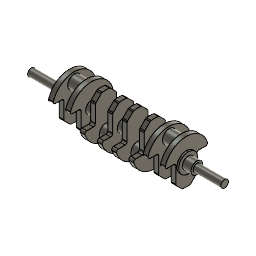
Four Cylinder Engine (Autodesk Fusion 360 archive; units mm, degrees)
design "Crank+Shaft"
Autodesk Fusion 360 part; units mm, degrees
sketch "Sketch1" plane through (0, 0, 0) normal (0, 1, 0) x (1, 0, 0)
  line L0 (0, 0) -> (0, -4)
  line L1 (0, -4) -> (29, -4)
  line L2 (29, -4) -> (29, -6.25)
  line L3 (29, -6.25) -> (38, -6.25)
  line L4 (38, -6.25) -> (38, -10)
  line L5 (38, -10) -> (40, -10)
  line L6 (40, -10) -> (40, 0)
  line L7 (40, 0) -> (0, 0)
  dimension "d1" = 40
  dimension "d2" = 8
  dimension "d3" = 9
  dimension "d4" = 2
  dimension "d5" = 12.5
  dimension "d6" = 20
  constraint coincident L0.start L7.end
  constraint vertical L0
  constraint perpendicular L0 L1
  constraint perpendicular L1 L2
  constraint perpendicular L2 L3
  constraint perpendicular L3 L4
  constraint perpendicular L4 L5
  constraint perpendicular L5 L6
  constraint perpendicular L6 L7
  measures "d1" distance of L6.end L0.start
  measures "d3" distance of L2.end L3.end
  measures "d4" distance of L4.end L5.end
revolve "Revolve1" add sketch "Sketch1" angle 360 about axis through (40, 0, 0) along (-1, 0, 0)
sketch "Sketch2" plane through (40, 0, 0) normal (1, 0, 0) x (0, 1, 0)
  circle A0 centre (0, 0) radius 10
  line L0 (-22.6495, 4) -> (-11, 4)
  line L1 (-11, 4) -> (-11, -16)
  line L2 (-11, -16) -> (-4.4308, -22.5692)
  line L3 (0, 0) -> (0, -30.8331) construction
  line L4 (0, -30.8331) -> (-15.3235, -23.6593) construction
  line L5 (22.6495, 4) -> (11, 4)
  line L6 (11, 4) -> (11, -16)
  line L7 (11, -16) -> (4.4308, -22.5692)
  arc A1 (-4.4308, -22.5692) -> (4.4308, -22.5692) centre (0, 0) ccw
  arc A2 (22.6495, 4) -> (-22.6495, 4) centre (0, 0) ccw
  dimension "d8" = 46
  dimension "d9" = 4
  dimension "d10" = 135
  dimension "d11" = 20
  dimension "d12" = 22
  dimension "d13" = 23
  constraint coincident A0.centre L3.start
  constraint horizontal L0
  constraint perpendicular L0 L1
  constraint vertical L3
  constraint symmetric L0.start L3 L5.start
  constraint symmetric L0.end L3 L5.end
  constraint symmetric L1.end L3 L6.end
  constraint symmetric L2.end L3 L7.end
  constraint concentric A1 A2
  measures "d8" diameter of A1
  measures "d9" distance of A0.centre L0
  measures "d10" angle of L1 L2
  measures "d11" distance of L0.end L1.end
  measures "d12" distance of L1 L6
  measures "d13" radius of A2
extrude "Extrude1" add sketch "Sketch2" along normal blind 5 contours A0 | L0 L1 L2 L5 L6 L7 A1 A2
fillet "Fillet1" radius 2 8 edges at (42.5, -22.6495, 4) (42.5, -11, -16) (42.5, -11, 4) (42.5, -4.4308, -22.5692) (42.5, 22.6495, 4) (42.5, 11, 4) (42.5, 11, -16) (42.5, 4.4308, -22.5692)
sketch "Sketch3" plane through (45, 0, 0) normal (1, 0, 0) x (0, 1, 0)
  arc A0 (3.7876, -22.686) -> (4.8725, -22.1275) centre (3.4583, -20.7133) ccw
  line L0 (4.8725, -22.1275) -> (10.4142, -16.5858)
  arc A1 (10.4142, -16.5858) -> (11, -15.1716) centre (9, -15.1716) ccw
  line L1 (11, -15.1716) -> (11, 2)
  arc A2 (13, 4) -> (11, 2) centre (13, 2) ccw
  line L2 (13, 4) -> (20.1246, 4)
  arc A3 (20.1246, 4) -> (22.0412, 6.5714) centre (20.1246, 6) ccw
  arc A4 (22.0412, 6.5714) -> (-22.0412, 6.5714) centre (0, 0) ccw
  arc A5 (-22.0412, 6.5714) -> (-20.1246, 4) centre (-20.1246, 6) ccw
  line L3 (-20.1246, 4) -> (-13, 4)
  arc A6 (-11, 2) -> (-13, 4) centre (-13, 2) ccw
  line L4 (-11, 2) -> (-11, -15.1716)
  arc A7 (-11, -15.1716) -> (-10.4142, -16.5858) centre (-9, -15.1716) ccw
  line L5 (-10.4142, -16.5858) -> (-4.8725, -22.1275)
  arc A8 (-4.8725, -22.1275) -> (-3.7876, -22.686) centre (-3.4583, -20.7133) ccw
  arc A9 (-3.7876, -22.686) -> (3.7876, -22.686) centre (0, 0) ccw
  circle A10 centre (0, 14) radius 7
  dimension "d18" = 14
  dimension "d19" = 14
  constraint vertical A4.centre A10.centre
  measures "d18" diameter of A10
  measures "d19" distance of A4.centre A10.centre
extrude "Extrude2" add sketch "Sketch3" along normal blind 13 contours A10
pattern_linear "R-Pattern1" count 2 spacing 18 along (1, 0, 0) of "Extrude1", "Fillet1"
sketch "Sketch4" plane through (63, 0, 0) normal (1, 0, 0) x (0, 1, 0)
  arc A0 (3.7876, -22.686) -> (4.8725, -22.1275) centre (3.4583, -20.7133) ccw
  line L0 (4.8725, -22.1275) -> (10.4142, -16.5858)
  arc A1 (10.4142, -16.5858) -> (11, -15.1716) centre (9, -15.1716) ccw
  line L1 (11, -15.1716) -> (11, 2)
  arc A2 (13, 4) -> (11, 2) centre (13, 2) ccw
  line L2 (13, 4) -> (20.1246, 4)
  arc A3 (20.1246, 4) -> (22.0412, 6.5714) centre (20.1246, 6) ccw
  arc A4 (22.0412, 6.5714) -> (-22.0412, 6.5714) centre (0, 0) ccw
  arc A5 (-22.0412, 6.5714) -> (-20.1246, 4) centre (-20.1246, 6) ccw
  line L3 (-20.1246, 4) -> (-13, 4)
  arc A6 (-11, 2) -> (-13, 4) centre (-13, 2) ccw
  line L4 (-11, 2) -> (-11, -15.1716)
  arc A7 (-11, -15.1716) -> (-10.4142, -16.5858) centre (-9, -15.1716) ccw
  line L5 (-10.4142, -16.5858) -> (-4.8725, -22.1275)
  arc A8 (-4.8725, -22.1275) -> (-3.7876, -22.686) centre (-3.4583, -20.7133) ccw
  arc A9 (-3.7876, -22.686) -> (3.7876, -22.686) centre (0, 0) ccw
  circle A10 centre (0, 0) radius 6.25
  dimension "d26" = 12.5
  constraint concentric A4 A10
  measures "d26" diameter of A10
extrude "Extrude3" add sketch "Sketch4" along normal blind 10 contours A10
sketch "Sketch5" plane through (73, 0, 0) normal (1, 0, 0) x (0, 1, 0)
  circle A0 centre (0, 0) radius 6.25
  line L0 (-22.6495, -4) -> (-11, -4)
  line L1 (-11, -4) -> (-11, 16)
  line L2 (-11, 16) -> (-4.4308, 22.5692)
  line L3 (0, 0) -> (0, 36.6926) construction
  line L4 (11, 16) -> (4.4308, 22.5692)
  line L5 (11, -4) -> (11, 16)
  line L6 (22.6495, -4) -> (11, -4)
  arc A1 (-22.6495, -4) -> (22.6495, -4) centre (0, 0) ccw
  arc A2 (4.4308, 22.5692) -> (-4.4308, 22.5692) centre (0, 0) ccw
  dimension "d29" = 46
  dimension "d30" = 135
  dimension "d31" = 20
  dimension "d32" = 11
  dimension "d33" = 4
  dimension "d34" = 23
  constraint coincident A0.centre L3.start
  constraint horizontal L0
  constraint perpendicular L0 L1
  constraint vertical L3
  constraint symmetric L0.start L3 L6.start
  constraint symmetric L0.end L3 L5.start
  constraint symmetric L1.end L3 L4.start
  constraint symmetric L2.end L3 L4.end
  constraint concentric A1 A2
  measures "d29" diameter of A1
  measures "d30" angle of L1 L2
  measures "d31" distance of L0.end L1.end
  measures "d32" distance of A0.centre L1
  measures "d33" vertical distance of A0.centre L0.start
  measures "d34" radius of A2
extrude "Extrude4" add sketch "Sketch5" along normal blind 5 contours A0 | L0 L1 L2 L4 L5 L6 A1 A2
fillet "Fillet2" radius 2 8 edges at (75.5, -11, 16) (75.5, -4.4308, 22.5692) (75.5, -11, -4) (75.5, -22.6495, -4) (75.5, 22.6495, -4) (75.5, 11, -4) (75.5, 11, 16) (75.5, 4.4308, 22.5692)
sketch "Sketch6" plane through (78, 0, 0) normal (1, 0, 0) x (0, 1, 0)
  arc A0 (4.8725, 22.1275) -> (3.7876, 22.686) centre (3.4583, 20.7133) ccw
  arc A1 (3.7876, 22.686) -> (-3.7876, 22.686) centre (0, 0) ccw
  arc A2 (-3.7876, 22.686) -> (-4.8725, 22.1275) centre (-3.4583, 20.7133) ccw
  line L0 (-4.8725, 22.1275) -> (-10.4142, 16.5858)
  arc A3 (-10.4142, 16.5858) -> (-11, 15.1716) centre (-9, 15.1716) ccw
  line L1 (-11, 15.1716) -> (-11, -2)
  arc A4 (-13, -4) -> (-11, -2) centre (-13, -2) ccw
  line L2 (-13, -4) -> (-20.1246, -4)
  arc A5 (-20.1246, -4) -> (-22.0412, -6.5714) centre (-20.1246, -6) ccw
  arc A6 (-22.0412, -6.5714) -> (22.0412, -6.5714) centre (0, 0) ccw
  arc A7 (22.0412, -6.5714) -> (20.1246, -4) centre (20.1246, -6) ccw
  line L3 (20.1246, -4) -> (13, -4)
  arc A8 (11, -2) -> (13, -4) centre (13, -2) ccw
  line L4 (11, -2) -> (11, 15.1716)
  arc A9 (11, 15.1716) -> (10.4142, 16.5858) centre (9, 15.1716) ccw
  line L5 (10.4142, 16.5858) -> (4.8725, 22.1275)
  circle A10 centre (0, -14) radius 7
  dimension "d39" = 14
  dimension "d40" = 14
  constraint vertical A1.centre A10.centre
  measures "d39" diameter of A10
  measures "d40" distance of A1.centre A10.centre
extrude "Extrude5" add sketch "Sketch6" along normal blind 13 contours A10
pattern_linear "R-Pattern2" count 2 spacing 18 along (1, 0, 0) of "Extrude4", "Fillet2"
sketch "Sketch7" plane through (96, 0, 0) normal (1, 0, 0) x (0, 1, 0)
  arc A0 (4.8725, 22.1275) -> (3.7876, 22.686) centre (3.4583, 20.7133) ccw
  arc A1 (3.7876, 22.686) -> (-3.7876, 22.686) centre (0, 0) ccw
  arc A2 (-3.7876, 22.686) -> (-4.8725, 22.1275) centre (-3.4583, 20.7133) ccw
  line L0 (-4.8725, 22.1275) -> (-10.4142, 16.5858)
  arc A3 (-10.4142, 16.5858) -> (-11, 15.1716) centre (-9, 15.1716) ccw
  line L1 (-11, 15.1716) -> (-11, -2)
  arc A4 (-13, -4) -> (-11, -2) centre (-13, -2) ccw
  line L2 (-13, -4) -> (-20.1246, -4)
  arc A5 (-20.1246, -4) -> (-22.0412, -6.5714) centre (-20.1246, -6) ccw
  arc A6 (-22.0412, -6.5714) -> (22.0412, -6.5714) centre (0, 0) ccw
  arc A7 (22.0412, -6.5714) -> (20.1246, -4) centre (20.1246, -6) ccw
  line L3 (20.1246, -4) -> (13, -4)
  arc A8 (11, -2) -> (13, -4) centre (13, -2) ccw
  line L4 (11, -2) -> (11, 15.1716)
  arc A9 (11, 15.1716) -> (10.4142, 16.5858) centre (9, 15.1716) ccw
  line L5 (10.4142, 16.5858) -> (4.8725, 22.1275)
  circle A10 centre (0, 0) radius 6.25
  dimension "d47" = 12.5
  constraint vertical A1.centre A6.centre
  constraint coincident A1.centre A6.centre
  measures "d47" diameter of A10
extrude "Extrude6" add sketch "Sketch7" along normal blind 5 contours A10
mirror "Mirror1" about plane through (101, 0, 0) normal (1, 0, 0) of bodies 1 merged
scale "Scale1" factor 25.4 about (45, -7, 14) bodies 1

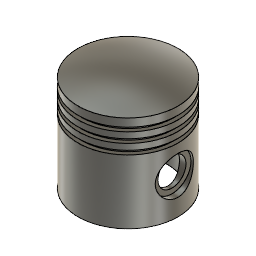
design "Piston (1)"
Autodesk Fusion 360 part; units mm, degrees
sketch "Sketch1" plane through (0, 0, 0) normal (0, 1, 0) x (1, 0, 0)
  line L0 (0, 0) -> (0, -786.4568) construction
  line L1 (0, -660.4) -> (0, -355.6)
  line L2 (0, -355.6) -> (254, -355.6)
  line L3 (254, -355.6) -> (254, 0)
  line L4 (254, 0) -> (317.5, 0)
  line L5 (317.5, 0) -> (317.5, -406.4)
  line L6 (317.5, -406.4) -> (292.1, -406.4)
  line L7 (292.1, -406.4) -> (292.1, -431.8)
  line L8 (292.1, -431.8) -> (317.5, -431.8)
  line L9 (317.5, -431.8) -> (317.5, -469.9)
  line L10 (317.5, -469.9) -> (292.1, -469.9)
  line L11 (292.1, -469.9) -> (292.1, -495.3)
  line L12 (292.1, -495.3) -> (317.5, -495.3)
  line L13 (317.5, -495.3) -> (317.5, -533.4)
  line L14 (317.5, -533.4) -> (292.1, -533.4)
  line L15 (292.1, -533.4) -> (292.1, -558.8)
  line L16 (292.1, -558.8) -> (317.5, -558.8)
  line L17 (317.5, -558.8) -> (317.5, -609.6)
  arc A0 (0, -660.4) -> (317.5, -609.6) centre (0, 357.1875) ccw
  line L18 (0, -660.4) -> (-554.1255, -660.4) construction
  dimension "d1" = 508
  dimension "d2" = 635
  dimension "d3" = 355.6
  dimension "d4" = 406.4
  dimension "d5" = 25.4
  dimension "d6" = 25.4
  dimension "d7" = 38.1
  dimension "d8" = 50.8
  dimension "d22" = 660.4
  constraint coincident L0.start origin
  constraint vertical L0
  constraint coincident L0 L1.start
  constraint coincident L0 L1.end
  constraint perpendicular L0 L2
  constraint perpendicular L2 L3
  constraint perpendicular L3 L4
  constraint perpendicular L4 L5
  constraint perpendicular L3 L6
  constraint perpendicular L6 L7
  constraint perpendicular L7 L8
  constraint perpendicular L8 L9
  constraint perpendicular L9 L10
  constraint perpendicular L10 L11
  constraint perpendicular L11 L12
  constraint perpendicular L12 L13
  constraint perpendicular L13 L14
  constraint perpendicular L14 L15
  constraint perpendicular L15 L16
  constraint perpendicular L16 L17
  constraint horizontal L0.start L3.end
  constraint vertical L5.end L8.end
  constraint vertical L9.end L12.end
  constraint vertical L13.end L16.end
  constraint equal L7 L11
  constraint equal L11 L15
  constraint equal L9 L13
  constraint vertical L7.end L10.end
  constraint vertical L11.end L14.end
  constraint perpendicular L0 L18
  constraint tangent A0 L18
  measures "d3" distance of L2.end L3.end
  measures "d4" distance of L4.end L5.end
  measures "d5" distance of L5.end L6.end
  measures "d6" distance of L6.end L7.end
  measures "d7" distance of L8.end L9.end
  measures "d8" distance of L16.end L17.end
  measures "d22" distance of L0.start L1.start
revolve "Revolve1" add sketch "Sketch1" angle 360 about axis through (0, 0, 0) along (0, 0, 1)
ref_plane "WorkPlane1" through (317.5, 0, 0) normal (1, 0, 0) x (0, 1, 0)
sketch "Sketch2" plane through (317.5, 0, 0) normal (1, 0, 0) x (0, 1, 0)
  circle A0 centre (0, 228.6) radius 120.65
  dimension "d13" = 241.3
  dimension "d14" = 228.6
  constraint vertical origin A0.centre
  measures "d13" diameter of A0
  measures "d14" distance of origin A0.centre
extrude "Extrude1" cut sketch "Sketch2" against normal blind 38.1
sketch "Sketch3" plane through (279.4, 0, 0) normal (1, 0, 0) x (0, 1, 0)
  circle A0 centre (0, 228.6) radius 120.65
  circle A1 centre (0, 228.6) radius 88.9
  dimension "d17" = 177.8
  constraint concentric A0 A1
  measures "d17" diameter of A1
extrude "Extrude2" cut sketch "Sketch3" against normal blind 127 contours A1
mirror "Mirror1" about plane through (0, 0, 0) normal (1, 0, 0) of "Extrude1", "Extrude2"

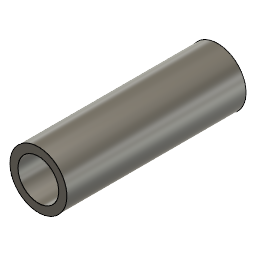
design "piston pin"
part number: 2026-06-25-16-27-55-743
Autodesk Fusion 360 part; units mm, degrees
sketch "Sketch1" plane through (0, 0, 0) normal (0, 0, 1) x (1, 0, 0)
  circle A0 centre (0, 0) radius 63.5
  circle A1 centre (0, 0) radius 88.9
  dimension "d2" = 127
  dimension "d3" = 177.8
  constraint coincident A0.centre A1.centre
  measures "d2" diameter of A0
  measures "d3" diameter of A1
extrude "Extrude1" add sketch "Sketch1" along normal blind 558.8

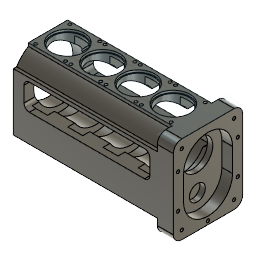
design "engine"
Autodesk Fusion 360 part; units mm, degrees
sketch "Sketch1" plane through (0, 0, 0) normal (1, 0, 0) x (0, 1, 0)
  line L0 (825.5, 1041.4) -> (-825.5, 1041.4)
  line L1 (-825.5, 1041.4) -> (-825.5, -1041.4)
  line L2 (-825.5, -1041.4) -> (825.5, -1041.4)
  line L3 (825.5, -1041.4) -> (825.5, 1041.4)
  line L4 (825.5, 1041.4) -> (-825.5, -1041.4) construction
  line L5 (-825.5, 1041.4) -> (825.5, -1041.4) construction
  dimension "d1" = 1651
  dimension "d2" = 2082.8
  constraint horizontal L0
  constraint perpendicular L0 L1
  constraint parallel L0 L2
  constraint parallel L1 L3
  constraint coincident L4 origin
  constraint coincident L5 origin
  measures "d1" distance of L0.start L0.end
  measures "d2" distance of L0.start L2.end
extrude "Extrude1" add sketch "Sketch1" along normal mid plane 3810
sketch "Sketch2" plane through (1905, 0, 0) normal (1, 0, 0) x (0, 1, 0)
  line L0 (825.5, -1041.4) -> (825.5, 1041.4)
  line L1 (825.5, 1041.4) -> (-825.5, 1041.4)
  line L2 (-825.5, 1041.4) -> (-825.5, -1041.4)
  line L3 (-825.5, -1041.4) -> (825.5, -1041.4)
  circle A0 centre (0, 279.4) radius 368.3
  dimension "d5" = 736.6
  dimension "d6" = 279.4
  constraint vertical origin A0.centre
  measures "d5" diameter of A0
  measures "d6" distance of origin A0.centre
extrude "Extrude2" cut sketch "Sketch2" against normal blind 3810 contours A0
sketch "Sketch3" plane through (1905, 0, 0) normal (1, 0, 0) x (0, 1, 0)
  circle A0 centre (0, 279.4) radius 368.3
  line L0 (825.5, -1041.4) -> (825.5, 1041.4)
  line L1 (825.5, 1041.4) -> (-825.5, 1041.4)
  line L2 (-825.5, 1041.4) -> (-825.5, -1041.4)
  line L3 (-825.5, -1041.4) -> (825.5, -1041.4)
  line L4 (-584.2, 279.4) -> (-584.2, -279.4)
  arc A1 (-584.2, -279.4) -> (584.2, -279.4) centre (0, -279.4) ccw
  line L5 (584.2, -279.4) -> (584.2, 279.4)
  arc A2 (584.2, 279.4) -> (-584.2, 279.4) centre (0, 279.4) ccw
  line L6 (0, 279.4) -> (0, -279.4) construction
  dimension "d9" = 584.2
  dimension "d10" = 558.8
  constraint tangent L4 A1
  constraint tangent A1 L5
  constraint parallel L4 L5
  constraint tangent L5 A2
  constraint tangent L4 A2
  constraint vertical L6
  constraint coincident A0.centre A2.centre
  measures "d9" radius of A2
  measures "d10" distance of A0.centre A1.centre
extrude "Extrude3" cut sketch "Sketch3" against normal blind 254 contours L4 A1 L5 A2
sketch "Sketch4" plane through (-1905, 0, 0) normal (-1, 0, 0) x (0, -1, 0)
  circle A0 centre (0, 279.4) radius 368.3
  line L0 (-825.5, 1041.4) -> (-825.5, -1041.4)
  line L1 (-825.5, -1041.4) -> (825.5, -1041.4)
  line L2 (825.5, -1041.4) -> (825.5, 1041.4)
  line L3 (825.5, 1041.4) -> (-825.5, 1041.4)
  circle A1 centre (0, 279.4) radius 590.55
  dimension "d13" = 1181.1
  constraint concentric A0 A1
  measures "d13" diameter of A1
extrude "Extrude4" cut sketch "Sketch4" against normal blind 3429 contours A1
sketch "Sketch5" plane through (-1905, 0, 0) normal (-1, 0, 0) x (0, -1, 0)
  circle A0 centre (0, 279.4) radius 590.55
  line L0 (-825.5, 1041.4) -> (-825.5, -1041.4)
  line L1 (-825.5, -1041.4) -> (825.5, -1041.4)
  line L2 (825.5, -1041.4) -> (825.5, 1041.4)
  line L3 (825.5, 1041.4) -> (-825.5, 1041.4)
  line L4 (-419.1, -1041.4) -> (-749.3, -685.8)
  line L5 (-749.3, -685.8) -> (-825.5, -685.8)
  line L6 (-825.5, 685.8) -> (-749.3, 685.8)
  arc A1 (-469.9, 965.2) -> (-749.3, 685.8) centre (-15.1369, 231.0369) ccw
  line L7 (-469.9, 965.2) -> (-469.9, 1041.4)
  line L8 (0, 0) -> (0, 1518.3954) construction
  line L9 (469.9, 965.2) -> (469.9, 1041.4)
  arc A2 (749.3, 685.8) -> (469.9, 965.2) centre (15.1369, 231.0369) ccw
  line L10 (825.5, 685.8) -> (749.3, 685.8)
  line L11 (419.1, -1041.4) -> (749.3, -685.8)
  line L12 (749.3, -685.8) -> (825.5, -685.8)
  dimension "d16" = 76.2
  dimension "d17" = 76.2
  dimension "d19" = 355.6
  dimension "d20" = 355.6
  dimension "d21" = 863.6
  dimension "d22" = 76.2
  dimension "d23" = 355.6
  dimension "d24" = 406.4
  constraint coincident L1 L4.start
  constraint coincident L0 L5.end
  constraint perpendicular L0 L5
  constraint coincident L0 L6.start
  constraint perpendicular L0 L6
  constraint coincident L3 L7.end
  constraint perpendicular L3 L7
  constraint coincident L8.start origin
  constraint parallel L2 L8
  constraint symmetric L4.start L8 L11.start
  constraint symmetric L4.end L8 L11.end
  constraint symmetric L5.end L8 L12.end
  constraint symmetric L6.start L8 L10.start
  constraint symmetric L6.end L8 A2.start
  constraint symmetric A1.start L8 L9.start
  constraint symmetric A1 L8 A2
  constraint symmetric L7.end L8 L9.end
  measures "d16" distance of A1.start L7.end
  measures "d17" distance of L6.start L6.end
  measures "d19" distance of L0.start L7.end
  measures "d20" distance of L0.start L6.start
  measures "d21" radius of A1
  measures "d22" distance of L4.end L5.end
  measures "d23" distance of L0.end L5.end
  measures "d24" distance of L0.end L4.start
extrude "Extrude5" cut sketch "Sketch5" against normal blind 3429 contours L0 L3 L6 A1 L7 | L0 L1 L4 L5 | L2 L3 L9 A2 L10 | L1 L2 L11 L12
sketch "Sketch6" plane through (0, 0, 1041.4) normal (0, 0, 1) x (-1, 0, 0)
  line L0 (-1524, 469.9) -> (-1524, 825.5)
  line L1 (-1524, 825.5) -> (-1905, 825.5)
  line L2 (-1905, 825.5) -> (-1905, -825.5)
  line L3 (-1905, -825.5) -> (-1524, -825.5)
  line L4 (-1524, -825.5) -> (-1524, -469.9)
  line L5 (-1524, -469.9) -> (1905, -469.9)
  line L6 (1905, -469.9) -> (1905, 469.9)
  line L7 (1905, 469.9) -> (-1524, 469.9)
  circle A0 centre (-1079.5, 0) radius 368.3
  circle A1 centre (-241.3, 0) radius 368.3
  circle A2 centre (596.9, 0) radius 368.3
  circle A3 centre (1435.1, 0) radius 368.3
  dimension "d27" = 736.6
  dimension "d28" = 825.5
  dimension "d31" = 2514.6
  dimension "d32" = 0
  constraint horizontal origin A0.centre
  measures "d27" diameter of A0
  measures "d28" distance of L2 A0.centre
extrude "Extrude6" cut sketch "Sketch6" against normal blind 762 contours A0 | A1 | A2 | A3
sketch "Sketch7" plane through (0, 0, 1041.4) normal (0, 0, 1) x (-1, 0, 0)
  circle A0 centre (596.9, 0) radius 368.3
  circle A1 centre (-241.3, 0) radius 368.3
  circle A2 centre (1435.1, 0) radius 368.3
  circle A3 centre (-1079.5, 0) radius 368.3
  line L0 (-1524, 469.9) -> (-1524, 825.5)
  line L1 (-1524, 825.5) -> (-1905, 825.5)
  line L2 (-1905, 825.5) -> (-1905, -825.5)
  line L3 (-1905, -825.5) -> (-1524, -825.5)
  line L4 (-1524, -825.5) -> (-1524, -469.9)
  line L5 (-1524, -469.9) -> (1905, -469.9)
  line L6 (1905, -469.9) -> (1905, 469.9)
  line L7 (1905, 469.9) -> (-1524, 469.9)
  circle A4 centre (-1079.5, 0) radius 393.7
  circle A5 centre (-241.3, 0) radius 393.7
  circle A6 centre (596.9, 0) radius 393.7
  circle A7 centre (1435.1, 0) radius 393.7
  dimension "d35" = 787.4
  dimension "d38" = 2514.6
  dimension "d39" = 0
  constraint concentric A3 A4
  measures "d35" diameter of A4
extrude "Extrude7" cut sketch "Sketch7" against normal blind 50.8 contours A4 | A5 | A6 | A7
sketch "Sketch8" plane through (0, 0, 0) normal (0, 1, 0) x (1, 0, 0)
  line L0 (1996.8796, -279.4) -> (-2336.7741, -279.4) construction
  line L1 (1270, -279.4) -> (914.4, -279.4)
  line L2 (914.4, -279.4) -> (914.4, -1016)
  line L3 (914.4, -1016) -> (1270, -1016)
  line L4 (1270, -1016) -> (1270, -279.4)
  line L5 (1905, -1041.4) -> (1905, 1041.4)
  dimension "d42" = 279.4
  dimension "d43" = 355.6
  dimension "d44" = 635
  dimension "d45" = 1473.2
  constraint horizontal L0
  constraint horizontal L1
  constraint vertical L2
  constraint horizontal L3
  constraint vertical L4
  constraint coincident L0 L1.start
  measures "d42" distance of origin L0
  measures "d43" distance of L2.end L3.end
  measures "d44" distance of L4 L5
revolve "Revolve1" cut sketch "Sketch8" angle 360 about axis through (1996.8796, 0, 279.4) along (-1, 0, 0)
pattern_linear "R-Pattern1" count 4 spacing 838.2 along (-1, 0, 0) of "Revolve1"
sketch "Sketch9" plane through (0, 0, 1041.4) normal (0, 0, 1) x (-1, 0, 0)
  circle A0 centre (596.9, 0) radius 393.7
  circle A1 centre (-241.3, 0) radius 393.7
  circle A2 centre (1435.1, 0) radius 393.7
  circle A3 centre (-1079.5, 0) radius 393.7
  line L0 (-1524, 469.9) -> (-1524, 825.5)
  line L1 (-1524, 825.5) -> (-1905, 825.5)
  line L2 (-1905, 825.5) -> (-1905, -825.5)
  line L3 (-1905, -825.5) -> (-1524, -825.5)
  line L4 (-1524, -825.5) -> (-1524, -469.9)
  line L5 (-1524, -469.9) -> (1905, -469.9)
  line L6 (1905, -469.9) -> (1905, 469.9)
  line L7 (1905, 469.9) -> (-1524, 469.9)
sketch "Sketch10" plane through (0, -825.5, 0) normal (0, -1, 0) x (1, 0, 0)
  line L0 (1524, 1041.4) -> (1524, 685.8)
  line L1 (1524, 685.8) -> (-1905, 685.8)
  line L2 (-1905, 685.8) -> (-1905, -685.8)
  line L3 (-1905, -685.8) -> (1524, -685.8)
  line L4 (1524, -685.8) -> (1524, -1041.4)
  line L5 (1524, -1041.4) -> (1905, -1041.4)
  line L6 (1905, -1041.4) -> (1905, 1041.4)
  line L7 (1905, 1041.4) -> (1524, 1041.4)
  line L8 (-1524, 596.9) -> (1219.2, 596.9)
  line L9 (1346.2, 469.9) -> (1346.2, 101.6)
  line L10 (1219.2, -25.4) -> (-1524, -25.4)
  line L11 (-1651, 101.6) -> (-1651, 469.9)
  line L12 (1524, 1041.4) -> (1905, 1041.4)
  arc A0 (-1524, 596.9) -> (-1651, 469.9) centre (-1524, 469.9) ccw
  arc A1 (-1651, 101.6) -> (-1524, -25.4) centre (-1524, 101.6) ccw
  arc A2 (1219.2, -25.4) -> (1346.2, 101.6) centre (1219.2, 101.6) ccw
  arc A3 (1346.2, 469.9) -> (1219.2, 596.9) centre (1219.2, 469.9) ccw
  dimension "d51" = 558.8
  dimension "d52" = 254
  dimension "d53" = 444.5
  dimension "d54" = 1016
  dimension "d55" = 127
  constraint horizontal L8
  constraint vertical L9
  constraint horizontal L10
  constraint vertical L11
  constraint tangent L8 A0
  constraint tangent L11 A0
  constraint tangent L10 A1
  constraint tangent L11 A1
  constraint equal A0 A1
  constraint tangent L9 A2
  constraint tangent L10 A2
  constraint equal A0 A2
  constraint tangent L8 A3
  constraint tangent L9 A3
  constraint equal A0 A3
  measures "d51" distance of L6 L9
  measures "d52" distance of L2 L11
  measures "d53" distance of L8 L12
  measures "d54" distance of L5 L10
  measures "d55" radius of A0
extrude "Extrude8" cut sketch "Sketch10" against normal blind 2286 contours L8 L9 L10 L11 A0 A1 A2 A3
sketch "Sketch11" plane through (0, 0, 1041.4) normal (0, 0, 1) x (-1, 0, 0)
  line L0 (-1435.1, -406.4) -> (-723.9, -406.4) construction
  line L1 (-723.9, -406.4) -> (-723.9, 406.4) construction
  line L2 (-723.9, 406.4) -> (-1435.1, 406.4) construction
  line L3 (-1435.1, 406.4) -> (-1435.1, -406.4) construction
  line L4 (-1435.1, -406.4) -> (-723.9, 406.4) construction
  line L5 (-723.9, -406.4) -> (-1435.1, 406.4) construction
  point P0 (-1079.5, 0)
  point P1 (-1079.5, 0)
  dimension "d58" = 711.2
  dimension "d59" = 812.8
  constraint horizontal L0
  constraint perpendicular L0 L1
  constraint parallel L0 L2
  constraint parallel L1 L3
  constraint coincident L4 P1
  constraint coincident L5 P1
  constraint coincident P1 P0
  measures "d58" distance of L0.start L0.end
  measures "d59" distance of L0.start L2.end
hole "Hole1" at (1435.1, 406.4, 1041.4) at (723.9, 406.4, 1041.4) at (723.9, -406.4, 1041.4) at (1435.1, -406.4, 1041.4) direction (0, 0, -1) diameter 69.85 depth 127 tip angle 118
pattern_linear "R-Pattern2" count 4 spacing 838.2 along (-1, 0, 0) of "Hole1"
sketch "Sketch12" plane through (1651, 0, 0) normal (1, 0, 0) x (0, 1, 0)
  circle A0 centre (0, 279.4) radius 368.3
  arc A1 (584.2, 279.4) -> (-584.2, 279.4) centre (0, 279.4) ccw
  line L0 (-584.2, 279.4) -> (-584.2, -279.4)
  arc A2 (-584.2, -279.4) -> (584.2, -279.4) centre (0, -279.4) ccw
  line L1 (584.2, -279.4) -> (584.2, 279.4)
  circle A3 centre (0, -508) radius 190.5
  dimension "d67" = 381
  dimension "d68" = 508
  constraint vertical origin A3.centre
  measures "d67" diameter of A3
  measures "d68" distance of origin A3.centre
extrude "Extrude9" cut sketch "Sketch12" against normal blind 127 contours A3
sketch "Sketch13" plane through (1905, 0, 0) normal (1, 0, 0) x (0, 1, 0)
  line L0 (-584.2, -279.4) -> (-584.2, 279.4)
  arc A0 (584.2, 279.4) -> (-584.2, 279.4) centre (0, 279.4) ccw
  line L1 (584.2, 279.4) -> (584.2, -279.4)
  arc A1 (-584.2, -279.4) -> (584.2, -279.4) centre (0, -279.4) ccw
  line L2 (825.5, -1041.4) -> (825.5, 1041.4)
  line L3 (825.5, 1041.4) -> (-825.5, 1041.4)
  line L4 (-825.5, 1041.4) -> (-825.5, -1041.4)
  line L5 (-825.5, -1041.4) -> (825.5, -1041.4)
  line L6 (0, 0) -> (0, 1626.6476) construction
  point P0 (-622.3, 838.2)
  point P1 (-711.2, 406.4)
  point P2 (-711.2, -406.4)
  point P3 (-622.3, -838.2)
  point P4 (0, -960.12)
  point P5 (622.3, 838.2)
  point P6 (711.2, 406.4)
  point P7 (711.2, -406.4)
  point P8 (622.3, -838.2)
  point P9 (0, -960.12)
  dimension "d71" = 711.2
  dimension "d72" = 812.8
  dimension "d73" = 406.4
  dimension "d74" = 960.12
  dimension "d75" = 203.2
  dimension "d76" = 431.8
  dimension "d77" = 203.2
  dimension "d78" = 431.8
  constraint coincident L6.start origin
  constraint vertical L6
  constraint vertical L6.start P9
  constraint vertical P1 P2
  constraint symmetric P0 L6 P5
  constraint symmetric P1 L6 P6
  constraint symmetric P2 L6 P7
  constraint symmetric P3 L6 P8
  constraint symmetric P9 L6 P4
  measures "d71" distance of P1 L6
  measures "d72" vertical distance of P1 P2
  measures "d73" vertical distance of L6.start P1
  measures "d74" distance of L6.start P9
  measures "d75" distance of L4 P3
  measures "d76" vertical distance of P2 P3
  measures "d77" distance of L4 P0
  measures "d78" vertical distance of P0 P1
hole "Hole2" at (1905, -622.3, 838.2) at (1905, -711.2, 406.4) at (1905, 711.2, 406.4) at (1905, 622.3, 838.2) at (1905, -711.2, -406.4) at (1905, -622.3, -838.2) at (1905, 0, -960.12) at (1905, 622.3, -838.2) at (1905, 711.2, -406.4) direction (-1, 0, 0) diameter 69.85 depth 127 tip angle 118 countersink diameter 76.835 countersink angle 82
fillet "Fillet1" radius 203.2 4 edges at (1714.5, -825.5, 1041.4) (1714.5, 825.5, 1041.4) (1714.5, -825.5, -1041.4) (1714.5, 825.5, -1041.4)
